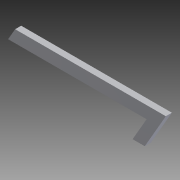
# Autodesk Inventor part: hook
Saved by Autodesk Inventor 2013 (Build 170138000, 138)
## iProperties
Created: 2013-01-20
Part Number: hook
Material: Aluminum 6061
Document SubType Name: Modeling
Designer: Arpan
Density: 1 g/cm^3
Author: Arpan
Autodesk Inventor part; units mm, degrees
ref_plane "YZ Plane" through (0, 0, 0) normal (1, 0, 0) x (0, 1, 0)
ref_plane "XZ Plane" through (0, 0, 0) normal (0, 1, 0) x (-1, 0, 0)
ref_plane "XY Plane" through (0, 0, 0) normal (0, 0, 1) x (1, 0, 0)
sketch "Sketch1" plane through (0, 0, 0) normal (0, 0, 1) x (1, 0, 0)
  line L0 (0, 0) -> (130.048, 0)
  line L1 (0, 0) -> (11.146, 19.3055)
  line L2 (87.9024, 12.7) -> (7.3323, 12.7)
  line L3 (87.9024, 12.7) -> (130.048, 12.7)
  line L4 (130.048, 12.7) -> (130.048, 0)
  line L5 (130.048, -25.4) -> (142.748, -25.4)
  line L6 (130.048, -25.4) -> (144.7127, 0)
  line L7 (142.748, -25.4) -> (164.745, 12.7)
  line L8 (144.7127, 0) -> (130.048, 0)
  line L9 (130.048, 12.7) -> (164.745, 12.7)
  dimension "d4" = 130.048
  dimension "d5" = 60
  dimension "d7" = 25.4
  dimension "d8" = 12.7
  dimension "d9" = 60
  dimension "d10" = 60
  dimension "d11" = 12.7
  constraints: 20 end point, 3 parallel, 1 collinear, 1 horizontal, 1 perpendicular, 1 point on line
  measures "d4" distance of L0.start L0.end
  measures "d5" angle of L0 L1
  measures "d7" distance of L0.end L5.start
  measures "d8" distance of L5.start L5.end
  measures "d9" angle of L6 L5
  measures "d10" angle of L5 L7
  measures "d11" distance between parallel lines of L2 L0
extrude "Extrusion1" add sketch "Sketch1" along normal blind 6.35
body "Solid1"
